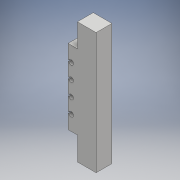
# Autodesk Inventor part: PiezaInferior
Saved by Autodesk Inventor 2017 (Build 210142000, 142)
## iProperties
Created: 2021-02-12
Part Number: PiezaInferior
Material: Generic
Document SubType Name: Modeling
Designer: USUARIO
Density: 1 g/cm^3
Appearance: Default
Author: USUARIO
Autodesk Inventor part; units mm, degrees
ref_plane "YZ Plane" through (0, 0, 0) normal (1, 0, 0) x (0, 1, 0)
ref_plane "XZ Plane" through (0, 0, 0) normal (0, 1, 0) x (-1, 0, 0)
ref_plane "XY Plane" through (0, 0, 0) normal (0, 0, 1) x (1, 0, 0)
sketch "Sketch3" plane through (0, 0, 0) normal (0, 1, 0) x (-1, 0, 0)
  line L0 (0, -390) -> (0, 0)
  line L1 (60, 0) -> (60, -75)
  line L2 (60, -75) -> (90, -75)
  line L3 (60, -390) -> (60, -315)
  line L4 (60, -315) -> (90, -315)
  line L5 (0, 0) -> (60, 0)
  line L6 (60, 0) -> (60, -75)
  line L7 (60, -75) -> (90, -75)
  line L8 (90, -75) -> (90, -315)
  line L9 (0, -390) -> (60, -390)
  circle A0 centre (80, -123) radius 7.5
  circle A1 centre (80, -171) radius 7.5
  circle A2 centre (80, -219) radius 7.5
  circle A3 centre (80, -267) radius 7.5
  dimension "d44" = 30
  dimension "d45" = 75
  dimension "d46" = 30
  dimension "d47" = 75
  dimension "d48" = 15
  dimension "d49" = 48
  dimension "d50" = 10
  dimension "d56" = 48
  constraints: 20 end point, 4 centre point, 2 collinear, 2 vertical, 1 horizontal, 6 other
  measures "d44" distance of L2.end L1.end
  measures "d45" distance of L1.end L1.start
  measures "d46" distance of L3.end L4.end
  measures "d47" distance of L3.start L3.end
  measures "d48" diameter of A0
  measures "d49" distance from line of L2 A0.centre
  measures "d50" distance from line of A0.centre L8
  measures "d56" distance of A0.centre A1.centre
extrude "Extrusion1" add sketch "Sketch3" along normal blind 50.8
sketch "Sketch6" plane through (0, 50.8, 0) normal (0, 1, 0) x (1, 0, 0)
  line L0 (-90, 315) -> (-90, 75) projected
  line L1 (-90, 120.5) -> (-87, 120.5)
  line L2 (-87, 120.5) -> (-87, 125.5)
  line L3 (-87, 125.5) -> (-90, 125.5)
  line L4 (-90, 125.5) -> (-90, 120.5)
  circle A0 centre (-80, 123) radius 7.5 projected
  line L5 (-87, 168.5) -> (-87, 173.5)
  line L6 (-87, 173.5) -> (-90, 173.5)
  line L7 (-90, 173.5) -> (-90, 168.5)
  line L8 (-90, 168.5) -> (-87, 168.5)
  line L9 (-87, 216.5) -> (-87, 221.5)
  line L10 (-87, 221.5) -> (-90, 221.5)
  line L11 (-90, 221.5) -> (-90, 216.5)
  line L12 (-90, 216.5) -> (-87, 216.5)
  line L13 (-87, 264.5) -> (-87, 269.5)
  line L14 (-87, 269.5) -> (-90, 269.5)
  line L15 (-90, 269.5) -> (-90, 264.5)
  line L16 (-90, 264.5) -> (-87, 264.5)
  point P0 (0, 0)
  dimension "d58" = 3
  dimension "d59" = 5
  dimension "d60" = 2.5
  dimension "d66" = 48
  constraints: 32 end point, 2 parallel, 1 horizontal, 1 perpendicular, 1 point on line, 1 vertical, 24 other
  measures "d58" distance of L3.end L2.end
  measures "d59" distance of L2.end L1.end
  measures "d60" distance from line of L1 A0.centre
  measures "d66" distance of L1.end L5.start
extrude "Extrusion3" cut sketch "Sketch6" against normal blind 50.8 contours L14 L13 L16 L0 | L3 A0 L1 L0 | L6 L5 L8 L0 | L10 L9 L12 L0 | L3 L2 L1 A0 picked at (-87.1506, 123.2826)
body "Solid1"
